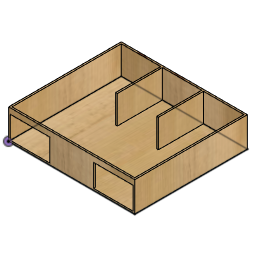
Optical Project Mechanical Design (Autodesk Fusion 360 design; units mm, degrees)
Autodesk Fusion 360 part; units mm, degrees
note: some values were not read from the file. Set by a fixed rule: which sketch regions a step uses.
sketch "Bottom " plane through (0, 0, 0) normal (0, 0, 1) x (1, 0, 0)
  line L0 (0, 0) -> (224, 0)
  line L1 (224, 0) -> (224, 200)
  line L2 (224, 200) -> (0, 200)
  line L3 (0, 200) -> (0, 0)
  dimension "d1" = 224
  dimension "d2" = 200
  constraint horizontal L0
  constraint vertical L1
  constraint horizontal L2
  constraint vertical L3
  constraint coincident L0.start L3.end
  measures "d1" distance of L0.start L0.end
  measures "d2" distance of L0.start L2.end
extrude "Extrude1" add sketch "Bottom " along normal blind 3
sketch "Left_Border" plane through (0, 0, 3) normal (0, 0, 1) x (-1, 0, 0)
  line L0 (0, -200) -> (0, 0)
  line L1 (0, 0) -> (-224, 0)
  line L2 (-224, 0) -> (-224, -200)
  line L3 (-224, -200) -> (0, -200)
  line L4 (0, 0) -> (-3, 0)
  line L5 (-3, 0) -> (-3, -200)
  line L6 (-3, -200) -> (0, -200)
  line L7 (0, -200) -> (0, 0)
  dimension "d5" = 3
  dimension "d6" = 200
  constraint horizontal L4
  constraint vertical L5
  constraint horizontal L6
  constraint vertical L7
  constraint coincident L0.end L1.start
  measures "d5" distance of L0.end L4.end
  measures "d6" distance of L0.end L0.start
sketch "Back_Border" plane through (0, 0, 3) normal (0, 0, 1) x (-1, 0, 0)
  line L0 (-3, -200) -> (-221, -200)
  line L1 (-221, -200) -> (-221, -197)
  line L2 (-221, -197) -> (-3, -197)
  line L3 (-3, -197) -> (-3, -200)
  dimension "d7" = 218
  constraint horizontal L0
  constraint vertical L1
  constraint horizontal L2
  constraint vertical L3
  measures "d7" distance of L0.start L0.end
sketch "Right_Border" plane through (0, 0, 3) normal (0, 0, 1) x (-1, 0, 0)
  line L0 (-224, -200) -> (-221, -200)
  line L1 (-221, -200) -> (-221, 0)
  line L2 (-221, 0) -> (-224, 0)
  line L3 (-224, 0) -> (-224, -200)
  dimension "d8" = 3
  dimension "d9" = 200
  constraint horizontal L0
  constraint vertical L1
  constraint horizontal L2
  constraint vertical L3
  measures "d8" distance of L0.start L0.end
  measures "d9" distance of L0.start L2.end
extrude "Extrude2" add sketch "Left_Border" along normal blind 50 contours L0 L1 L3 L4 L5 L6 L7
extrude "Extrude3" add sketch "Back_Border" along normal blind 50
extrude "Extrude4" add sketch "Right_Border" along normal blind 50
sketch "limi_1" plane through (0, 0, 3) normal (0, 0, 1) x (-1, 0, 0)
  line L0 (-221, -197) -> (-3, -197)
  line L1 (-3, -197) -> (-3, 0)
  line L2 (-3, 0) -> (-221, 0)
  line L3 (-73, -197) -> (-73, -117)
  line L4 (-73, -197) -> (-76, -197)
  line L5 (-76, -197) -> (-76, -117)
  line L6 (-76, -117) -> (-73, -117)
  line L7 (-221, 0) -> (-221, -197)
  dimension "d17" = 80
  dimension "d18" = 3
  dimension "d19" = 80
  constraint coincident L0 L3.start
  constraint perpendicular L0 L3
  constraint horizontal L4
  constraint vertical L5
  constraint horizontal L6
  measures "d17" distance of L3.start L3.end
  measures "d18" distance of L3.start L4.end
  measures "d19" distance of L3.start L3.end
extrude "Extrude5" add sketch "limi_1" along normal blind 50 contours L0 L3 L4 L5 L6
sketch "limi_2" plane through (0, 0, 3) normal (0, 0, 1) x (-1, 0, 0)
  line L0 (-73, -117) -> (-73, -197)
  line L1 (-73, -197) -> (-3, -197)
  line L2 (-3, -197) -> (-3, 0)
  line L3 (-3, 0) -> (-221, 0)
  line L4 (-76, -197) -> (-76, -117)
  line L5 (-76, -117) -> (-73, -117)
  line L6 (-146, -197) -> (-149, -197)
  line L7 (-149, -197) -> (-149, -117)
  line L8 (-149, -117) -> (-146, -117)
  line L9 (-146, -117) -> (-146, -197)
  line L10 (-221, 0) -> (-221, -197)
  line L11 (-221, -197) -> (-76, -197)
  dimension "d22" = 70
  dimension "d24" = 3
  dimension "d25" = 80
  constraint horizontal L6
  constraint vertical L7
  constraint horizontal L8
  constraint vertical L9
  measures "d22" distance of L4.start L6.start
  measures "d24" distance of L6.start L6.end
  measures "d25" distance of L6.start L8.end
extrude "Extrude6" add sketch "limi_2" along normal blind 50 contours L6 L7 L8 L9 L11
sketch "Large_Front_Side" plane through (0, 0, 3) normal (0, 0, 1) x (-1, 0, 0)
  line L0 (-149, -197) -> (-149, -117)
  line L1 (-149, -117) -> (-146, -117)
  line L2 (-146, -117) -> (-146, -197)
  line L3 (-146, -197) -> (-76, -197)
  line L4 (-76, -197) -> (-76, -117)
  line L5 (-76, -117) -> (-73, -117)
  line L6 (-73, -117) -> (-73, -197)
  line L7 (-73, -197) -> (-3, -197)
  line L8 (-3, -197) -> (-3, 0)
  line L9 (-3, 0) -> (-221, 0)
  line L10 (-221, 0) -> (-221, -197)
  line L11 (-221, -197) -> (-149, -197)
  line L12 (-3, 0) -> (-73, 0)
  line L13 (-221, 0) -> (-151, 0)
  line L14 (-73, 0) -> (-151, 0)
  line L15 (-151, 0) -> (-151, -3)
  line L16 (-151, -3) -> (-73, -3)
  line L17 (-73, -3) -> (-73, 0)
  dimension "d28" = 70
  dimension "d29" = 70
  dimension "d30" = 3
  constraint coincident L8.end L9.start
  constraint perpendicular L8 L12
  constraint coincident L9.end L10.start
  constraint perpendicular L10 L13
  constraint horizontal L14
  constraint vertical L15
  constraint horizontal L16
  constraint vertical L17
  measures "d28" distance of L8.end L12.end
  measures "d29" distance of L9.end L13.end
  measures "d30" distance of L12.end L16.end
extrude "Extrude7" add sketch "Large_Front_Side" along normal blind 50 contours L9 L14 L15 L16 L17
sketch "Sketch8" plane through (73, 0, 0) normal (-1, 0, 0) x (0, -1, 0)
  line L0 (-3, 3) -> (0, 3)
  line L1 (0, 3) -> (0, 53)
  line L2 (0, 53) -> (-3, 53)
  line L3 (-3, 53) -> (-3, 3)
  line L4 (-3, 53) -> (0, 53)
  line L5 (0, 53) -> (0, 43)
  line L6 (0, 43) -> (-3, 43)
  line L7 (-3, 43) -> (-3, 53)
  dimension "d33" = 3
  dimension "d34" = 10
  constraint horizontal L4
  constraint vertical L5
  constraint horizontal L6
  constraint vertical L7
  constraint coincident L2.end L3.start
  measures "d33" distance of L2.end L1.end
  measures "d34" distance of L2.end L6.end
extrude "Extrude8" add sketch "Sketch8" along normal blind 70 contours L1 L2 L3 L4 L5 L6 L7
sketch "Sketch9" plane through (151, 0, 0) normal (1, 0, 0) x (0, 1, 0)
  line L0 (0, 3) -> (3, 3)
  line L1 (3, 3) -> (3, 53)
  line L2 (3, 53) -> (0, 53)
  line L3 (0, 53) -> (0, 3)
  line L4 (0, 53) -> (3, 53)
  line L5 (3, 53) -> (3, 43)
  line L6 (3, 43) -> (0, 43)
  line L7 (0, 43) -> (0, 53)
  dimension "d37" = 3
  dimension "d38" = 10
  constraint horizontal L4
  constraint vertical L5
  constraint horizontal L6
  constraint vertical L7
  constraint coincident L2.end L3.start
  measures "d37" distance of L2.end L1.end
  measures "d38" distance of L2.end L6.end
extrude "Extrude9" add sketch "Sketch9" along normal blind 70 contours L1 L2 L3 L4 L5 L6 L7
equation "d7 = 221 mm - 3 mm"
